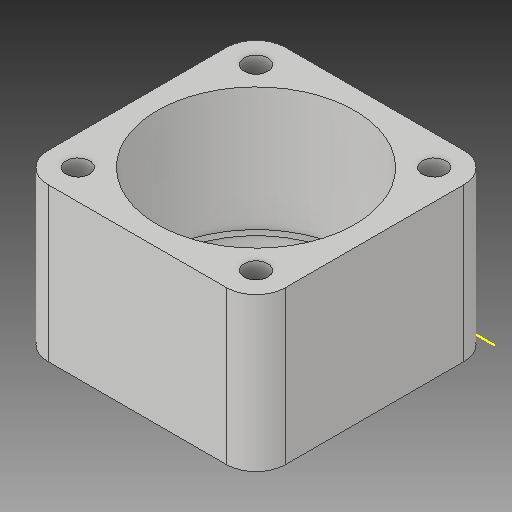
# Autodesk Inventor part: frame
Saved by Autodesk Inventor 2018 (Build 220112000, 112)
## iProperties
Created: 2020-03-23
Part Number: frame
Material: Generic
Document SubType Name: Modeling
Designer: emile
Density: 1 g/cm^3
Appearance: Default
Author: emile
Autodesk Inventor part; units mm, degrees
ref_plane "YZ Plane" through (0, 0, 0) normal (1, 0, 0) x (0, 1, 0)
ref_plane "XZ Plane" through (0, 0, 0) normal (0, 1, 0) x (-1, 0, 0)
ref_plane "XY Plane" through (0, 0, 0) normal (0, 0, 1) x (1, 0, 0)
sketch "Sketch1" plane through (0, 0, 0) normal (0, 1, 0) x (-1, 0, 0)
  circle A0 centre (0, 0) radius 42.2275
  circle A1 centre (0, 0) radius 50.8
  line L0 (0, 50.8) -> (-50.8, 50.8)
  line L1 (-50.8, 50.8) -> (-50.8, -50.8)
  line L2 (-50.8, -50.8) -> (0, -50.8)
  circle A2 centre (0, 0) radius 39.0525
  circle A3 centre (0, 0) radius 35.8775
  circle A4 centre (0, 0) radius 32.7025
  circle A5 centre (0, 0) radius 29.5275
  circle A6 centre (0, 0) radius 26.3525
  circle A7 centre (0, 0) radius 23.1775
  circle A8 centre (0, 0) radius 20.0025
  circle A9 centre (0, 0) radius 16.8275
  circle A10 centre (0, 0) radius 13.6525
  circle A11 centre (0, 0) radius 10.4775
  line L3 (0, 3.175) -> (42.2275, 3.175)
  line L4 (42.2275, 3.175) -> (42.2275, -3.175)
  line L5 (42.2275, -3.175) -> (0, -3.175)
  line L6 (0, -3.175) -> (0, 3.175)
  point P0 (42.2275, 0)
  dimension "d0" = 84.455
  dimension "d2" = 50.8
  dimension "d3" = 50.8
  dimension "d6" = 3.175
  dimension "d7" = 3.175
  dimension "d8" = 3.175
  dimension "d9" = 3.175
  dimension "d10" = 3.175
  dimension "d11" = 3.175
  dimension "d12" = 3.175
  dimension "d13" = 3.175
  dimension "d14" = 3.175
  dimension "d15" = 3.175
  dimension "d16" = 6.35
  constraints: 14 end point, 13 coincident, 11 centre point, 3 perpendicular, 2 horizontal, 2 midpoint, 2 parallel, 2 point on circle, 2 tangent, 1 horizontal alignment, 2 other
  measures "d2" distance from line of L0 point (0, 0)
  measures "d3" distance from line of point (0, 0) L2
  measures "d7" radial gap between concentric circles of A2 A3
  measures "d8" radial gap between concentric circles of A3 A4
  measures "d9" radial gap between concentric circles of A4 A5
  measures "d10" radial gap between concentric circles of A5 A6
  measures "d11" radial gap between concentric circles of A6 A7
  measures "d12" radial gap between concentric circles of A7 A8
  measures "d13" radial gap between concentric circles of A8 A9
  measures "d14" radial gap between concentric circles of A9 A10
  measures "d15" radial gap between concentric circles of A10 A11
  measures "d16" distance between parallel lines of L5 L3
extrude "Extrusion1" add sketch "Sketch1" along normal blind 52.8574
extrude "Extrusion2" add sketch "Sketch1" against normal blind 12.7 contours A0 L5 A2 L3 | L4 L5 A0 | A0 L3 L4 | A2 L5 A3 L3 | A3 L5 A4 L3 | A4 L5 A5 L3 | A5 L5 A6 L3 | A6 L5 A7 L3 | A7 L5 A8 L3 | A8 L5 A9 L3 | A9 L5 A10 L3 | A10 L5 A11 L3 | A11 L5 L6 L3 picked at (40.0087, 2.8227) picked at (36.825, 2.8227) picked at (33.6395, 2.8228) picked at (30.4519, -2.823) picked at (27.2613, 2.8232) picked at (24.0666, 2.8235) picked at (20.8659, -2.8239) picked at (17.6557, 2.8246) picked at (14.4297, -2.8258) picked at (11.3886, 1.7788) picked at (3.4925, 0)
extrude "Extrusion3" add sketch "Sketch1" against normal blind 12.7 contours A0 L5 A2 L3 | L3 A2 L5 A0 | L3 L6 L5 A11 | A11 L5 L6 L3
pattern_circular "Circular Pattern1" count 4 over 360 about axis through (0, 0, 0) along (0, -1, 0) of "Extrusion2"
extrude "Extrusion4" add sketch "Sketch1" against normal up to surface (12.7 mm away)
sketch "Sketch4" plane through (0, 52.8574, 0) normal (0, 1, 0) x (1, 0, 0)
  line L0 (0, -50.8) -> (50.8, -50.8) projected
  line L1 (50.8, -50.8) -> (50.8, 50.8) projected
  line L2 (50.8, 50.8) -> (0, 50.8) projected
  arc A0 (0, 50.8) -> (0, -50.8) centre (0, 0) ccw projected
  arc A1 (-42.108, -3.175) -> (-42.108, 3.175) centre (0, 0) ccw projected
  line L3 (-42.108, -3.175) -> (-42.2275, -3.175) projected
  line L4 (-42.2275, -3.175) -> (-42.2275, 3.175) projected
  line L5 (-42.2275, 3.175) -> (-42.108, 3.175) projected
sketch "Sketch5" plane through (0, 0, 0) normal (0, 1, 0) x (0, 0, -1)
  circle A0 centre (0, 0) radius 7.9375
  dimension "d30" = 15.875
  constraints: 1 centre point, 1 coincident
  measures "d30" diameter of A0
extrude "Extrusion7" cut sketch "Sketch5" against normal blind 5.334
sketch "Sketch6" plane through (0, -5.334, 0) normal (0, 1, 0) x (1, 0, 0)
  circle A0 centre (0, 0) radius 6.6675
  dimension "d33" = 13.335
  constraints: 1 centre point, 1 coincident
  measures "d33" diameter of A0
extrude "Extrusion8" cut sketch "Sketch6" against normal through all
sketch "Sketch7" plane through (0, 52.8574, 0) normal (0, 1, 0) x (1, 0, 0)
  point P0 (0, 0)
fillet "Fillet1" radius 3.175 14 edges at (-3.175, -6.35, -38.9232) (-38.9232, -6.35, -3.175) (-3.175, -6.35, -9.9849) (-9.9849, -6.35, -3.175) (-9.9849, -6.35, 3.175) (-38.9232, -6.35, 3.175) (-3.175, -6.35, 38.9232) (-3.175, -6.35, 9.9849) (3.175, -6.35, 9.9849) (9.9849, -6.35, 3.175) (38.9232, -6.35, 3.175) (38.9232, -6.35, -3.175) (3.175, -6.35, -38.9232) (3.175, -6.35, 38.9232)
sketch "Sketch11" plane through (0, 0, 0) normal (0, 1, 0) x (1, 0, 0)
  arc A0 (-42.108, -3.175) -> (-42.108, 3.175) centre (0, 0) ccw projected
  arc A1 (-42.108, 3.175) -> (-42.108, -3.175) centre (0, 0) ccw
  line L0 (-42.2275, 3.175) -> (-42.2275, -3.175) projected
  line L1 (-42.108, -3.175) -> (-42.2275, -3.175)
  line L2 (-42.2275, 3.175) -> (-42.108, 3.175)
  constraints: 4 end point, 2 point on circle, 1 centre point, 1 parallel, 1 perpendicular, 1 tangent
extrude "Extrusion11" add sketch "Sketch11" along normal up to surface (52.8574 mm away) contours L1 L0 A1 | A1 L0 L2
sketch "Sketch12" plane through (0, 52.8574, 0) normal (0, 1, 0) x (1, 0, 0)
  arc A0 (0, 50.8) -> (0, -50.8) centre (0, 0) ccw projected
  line L0 (0, -50.8) -> (-50.8, -50.8)
  line L1 (-50.8, -50.8) -> (-50.8, 0)
  constraints: 4 end point, 2 tangent, 1 horizontal, 1 perpendicular, 1 point on circle
extrude "Extrusion12" add sketch "Sketch12" against normal up to surface (65.5574 mm away)
sketch "Sketch13" plane through (0, -12.7, 0) normal (0, -1, 0) x (1, 0, 0)
  point P0 (-38.1, 38.1)
  point P1 (38.1, 38.1)
  point P2 (38.1, -38.1)
  point P3 (-38.1, -38.1)
hole "Hole1" at (-38.1, -12.7, 38.1) at (38.1, -12.7, 38.1) at (38.1, -12.7, -38.1) at (-38.1, -12.7, -38.1) direction (0, 1, 0) diameter 10.0838 depth 65.5574
sketch "Sketch17" plane through (0, -12.7, 0) normal (0, -1, 0) x (1, 0, 0)
  line L0 (50.8, -50.8) -> (0, -50.8) projected
  line L1 (0, -50.8) -> (-50.8, -50.8)
  line L2 (-50.8, -50.8) -> (-50.8, 0)
  circle A0 centre (-38.1, -38.1) radius 5.0419
  circle A1 centre (38.1, -38.1) radius 5.0419 projected
  circle A2 centre (38.1, 38.1) radius 5.0419 projected
  circle A3 centre (-38.1, 38.1) radius 5.0419 projected
  arc A4 (-50.8, 0) -> (0, -50.8) centre (0, 0) ccw projected
  constraints: 4 end point, 1 centre point, 1 equal radius, 1 horizontal, 1 horizontal alignment, 1 perpendicular, 1 vertical alignment
extrude "Extrusion15" add sketch "Sketch17" against normal up to surface (65.5574 mm away) contours L1 L2 A4 A0 | A0 A4 picked at (-37.6782, -37.9609)
extrude "Extrusion16" cut sketch "Sketch17" against normal through all contours A4 A0 | A0 A4
fillet "Fillet3" radius 12.7 4 edges at (-50.8, 20.0787, -50.8) (-50.8, 20.0787, 50.8) (50.8, 20.0787, 50.8) (50.8, 20.0787, -50.8)
equation "\"d3\" = d2"
equation "\"d8\" = d7"
equation "\"d9\" = d8"
equation "\"d10\" = d9"
equation "\"d11\" = d10"
equation "\"d12\" = d11"
equation "\"d13\" = d10"
equation "\"d14\" = d13"
equation "\"d15\" = d13"
body "Solid1"
